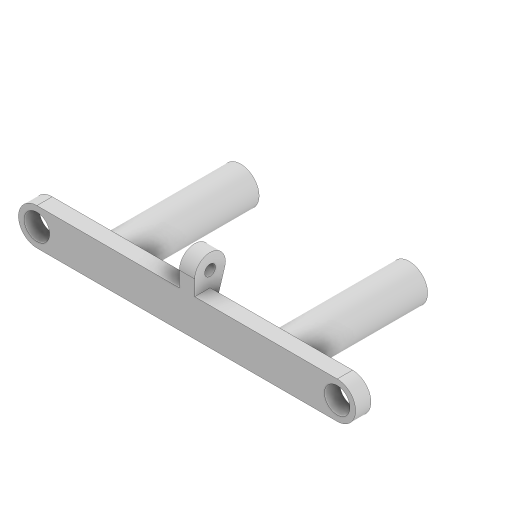
# Autodesk Inventor part: Support slider
Saved by Autodesk Inventor 2024 (Build 280153000, 153)
## iProperties
Created: 2025-04-26
Part Number: Support slider
Material: Generic
Document SubType Name: Modeling
Designer: Binara
Density: 1 g/cm^3
Appearance: Default
Author: Binara
## iProperties of the stored document Support slider_3DPrint.ipt
Created: 2025-04-26
Part Number: Support slider_3DPrint
Material: Generic
Document SubType Name: Modeling
Designer: Binara
Density: 1 g/cm^3
Appearance: Default
Author: Binara
Autodesk Inventor part; units mm, degrees
ref_plane "YZ Plane" through (0, 0, 0) normal (1, 0, 0) x (0, 1, 0)
ref_plane "XZ Plane" through (0, 0, 0) normal (0, 1, 0) x (-1, 0, 0)
ref_plane "XY Plane" through (0, 0, 0) normal (0, 0, 1) x (1, 0, 0)
sketch "Sketch1" plane through (0, 0, 0) normal (0, 0, 1) x (1, 0, 0)
  line L0 (-49, 0) -> (49, 0) construction
  line L1 (-49, -6) -> (49, -6)
  line L2 (49, 6) -> (-49, 6)
  arc A0 (-49, 6) -> (-49, -6) centre (-49, 0) ccw
  arc A1 (49, -6) -> (49, 6) centre (49, 0) ccw
  circle A2 centre (49, 0) radius 4.15
  circle A3 centre (-49, 0) radius 4.15
  point P0 (0, 0)
  dimension "d0" = 49
  dimension "d1" = 12
  dimension "d2" = 8.3
  dimension "d3" = 8.3
  constraints: 8 end point, 4 centre point, 4 point on circle, 4 tangent, 2 coincident, 1 horizontal, 1 midpoint, 1 parallel
  measures "d0" distance of point (0, 0) L0.end
  measures "d1" diameter of A1
  measures "d2" diameter of A2
  measures "d3" diameter of A3
extrude "Extrusion1" add sketch "Sketch1" along normal blind 5
sketch "Sketch2" plane through (0, 0, 0) normal (1, 0, 0) x (0, 1, 0)
  circle A0 centre (11, 0) radius 1.75
  circle A1 centre (11, 0) radius 5
  line L0 (6, 5) -> (-6, 5) projected
  line L1 (6, 5) -> (11, 5)
  line L2 (9.5294, -4.7788) -> (-6, 0)
  line L3 (-6, 0) -> (6, 0) projected
  line L4 (6, 0) -> (6, 5) projected
  line L5 (-6, 5) -> (6, 5) projected
  line L6 (-6, 0) -> (-6, 5) projected
  line L7 (6, 0) -> (6, 5) projected
  point P0 (0, 0)
  point P1 (-6, 0)
  dimension "d6" = 3.5
  dimension "d7" = 10
  constraints: 4 end point, 4 tangent, 2 centre point, 2 coincident, 2 point on circle
  measures "d6" diameter of A0
  measures "d7" diameter of A1
extrude "Extrusion2" add sketch "Sketch2" along normal mid plane 5 contours A1 | A1 L4 L1 | L2 L3 A1
sketch "Sketch3" plane through (0, 0, 0) normal (0, 0, -1) x (-1, 0, 0)
  circle A0 centre (-27.5, 0) radius 6
  line L0 (-49, 6) -> (-2.5, 6) projected
  line L1 (2.5, -6) -> (-2.5, -6) projected
  line L2 (0, -6) -> (0, -9.8516)
  line L3 (-2.5, -6) -> (-49, -6) projected
  line L4 (-2.5, -6) -> (-2.5, 9.5294) projected
  circle A1 centre (27.5, 0) radius 6
  point P0 (0, 0)
  dimension "d10" = 25
  constraints: 2 centre point, 2 end point, 2 tangent, 1 midpoint, 1 symmetric about line, 1 vertical, 1 other
  measures "d10" distance from line of L4 A0.centre
extrude "Extrusion3" add sketch "Sketch3" along normal blind 40 contours A0 | A1
body "Solid1"
